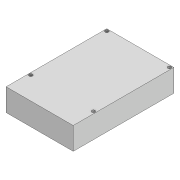
# Autodesk Inventor part: Raspberry_Dummy
Saved by Autodesk Inventor 2020 (Build 240168000, 168)
## iProperties
Created: 2021-06-30
Part Number: Raspberry_Dummy
Material: Generisch
Document SubType Name: Modeling
Designer: Julian Uhl
Density: 1 g/cm^3
Appearance: Vorgabe
Author: Julian Uhl
Autodesk Inventor part; units mm, degrees
ref_plane "YZ Plane" through (0, 0, 0) normal (1, 0, 0) x (0, 1, 0)
ref_plane "XZ Plane" through (0, 0, 0) normal (0, 1, 0) x (-1, 0, 0)
ref_plane "XY Plane" through (0, 0, 0) normal (0, 0, 1) x (1, 0, 0)
sketch "Skizze1" plane through (0, 0, 0) normal (0, 1, 0) x (-1, 0, 0)
  line L0 (0, 0) -> (-60, 0)
  line L1 (-60, 0) -> (-60, -90)
  line L2 (-60, -90) -> (0, -90)
  line L3 (0, -90) -> (0, 0)
  dimension "d0" = 60
  dimension "d1" = 90
  constraints: 8 end point, 2 parallel, 1 horizontal, 1 perpendicular
  measures "d0" distance of L2.end L1.end
  measures "d1" distance of L1.end L0.end
extrude "Extrusion1" add sketch "Skizze1" along normal blind 20
sketch "Skizze2" plane through (0, 20, 0) normal (0, 1, 0) x (1, 0, 0)
  line L0 (60, 0) -> (60, 90) projected
  line L1 (60, 90) -> (0, 90) projected
  line L2 (0, 90) -> (0, 0) projected
  line L3 (0, 0) -> (60, 0) projected
  point P0 (58, 88)
  point P1 (2, 88)
  point P2 (2, 20)
  point P3 (58, 20)
  dimension "d4" = 2
  dimension "d5" = 2
  dimension "d6" = 2
  dimension "d7" = 2
  dimension "d8" = 2
  dimension "d9" = 2
  dimension "d10" = 20
  dimension "d11" = 20
  measures "d4" distance from line of L0 point (58, 88)
  measures "d5" distance from line of L1 point (58, 88)
  measures "d6" distance from line of L1 point (2, 88)
  measures "d7" distance from line of L2 point (2, 88)
  measures "d8" distance from line of L2 point (2, 20)
  measures "d9" distance from line of L0 point (58, 20)
  measures "d10" distance from line of L3 point (58, 20)
  measures "d11" distance from line of L3 point (2, 20)
hole "Bohrung1" at (58, 20, -88) at (58, 20, -20) at (2, 20, -88) at (2, 20, -20) direction (0, -1, 0) diameter 3 end through all
